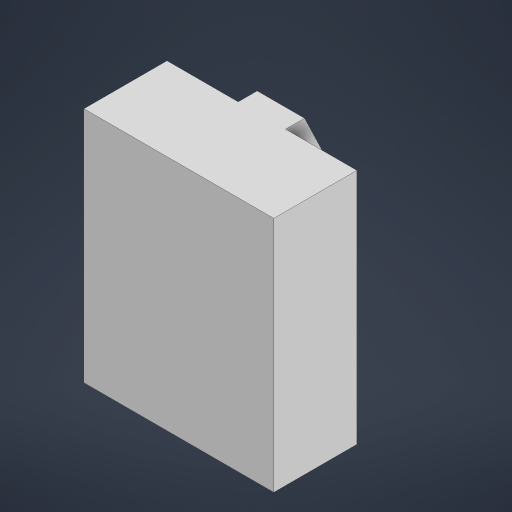
# Autodesk Inventor part: prueba
Saved by Autodesk Inventor 2024.1 (Build 281209000, 209)
## iProperties
Created: 2023-07-19
Part Number: prueba
Material: Generic
Document SubType Name: Modeling
Designer: LabTel_Admin
Density: 1 g/cm^3
Appearance: Default
Author: LabTel_Admin
Autodesk Inventor part; units mm, degrees
ref_plane "YZ Plane" through (0, 0, 0) normal (1, 0, 0) x (0, 1, 0)
ref_plane "XZ Plane" through (0, 0, 0) normal (0, 1, 0) x (-1, 0, 0)
ref_plane "XY Plane" through (0, 0, 0) normal (0, 0, 1) x (1, 0, 0)
sketch "Sketch1" plane through (0, 0, 0) normal (0, 1, 0) x (-1, 0, 0)
  line L0 (0, 0) -> (-8, 0)
  line L1 (-8, 0) -> (-8, -3.5)
  line L2 (-8, -3.5) -> (0, -3.5)
  line L3 (0, -3.5) -> (0, 0)
  dimension "d0" = 8
  dimension "d1" = 3.5
  constraints: 8 end point, 2 parallel, 1 horizontal, 1 perpendicular
  measures "d0" distance of L2.end L1.end
  measures "d1" distance of L1.end L0.end
extrude "Extrusion1" add sketch "Sketch1" along normal blind 10
sketch "Sketch2" plane through (8, 0, -3.5) normal (0, 0, -1) x (-1, 0, 0)
  line L0 (0, 10) -> (8, 10) projected
  line L1 (3, 10) -> (5, 10)
  line L2 (5, 10) -> (5, 5)
  line L3 (5, 5) -> (3, 5)
  line L4 (3, 5) -> (3, 10)
  line L5 (8, 0) -> (8, 10) projected
  dimension "d4" = 2
  dimension "d5" = 5
  dimension "d6" = 3
  constraints: 8 end point, 2 parallel, 1 horizontal, 1 perpendicular, 1 point on line
  measures "d4" distance of L2.end L3.end
  measures "d5" distance of L1.end L2.end
  measures "d6" distance between parallel lines of L5 L2
extrude "Extrusion2" add sketch "Sketch2" along normal blind 3
sketch "Sketch3" plane through (5, 5, -3.5) normal (1, 0, 0) x (0, 0, -1)
  line L0 (0, 5) -> (3, 5) projected
  line L1 (0.8, 5) -> (3, 0.4)
  line L2 (3, 0) -> (3, 5) projected
  line L3 (0, -5) -> (0, 5) projected
  line L4 (0, 0) -> (3, 0) projected
  line L5 (0.8, 5) -> (3, 5)
  line L6 (3, 0.4) -> (3, 5)
  point P0 (-3.5, -5)
  dimension "d9" = 0.8
  dimension "d10" = 0.4
  constraints: 6 end point, 2 collinear, 2 point on line
  measures "d9" distance from line of L3 L1.start
  measures "d10" distance from line of L4 L1.end
extrude "Extrusion3" cut sketch "Sketch3" against normal through all contours L0 L2 L1
body "Solid1"
